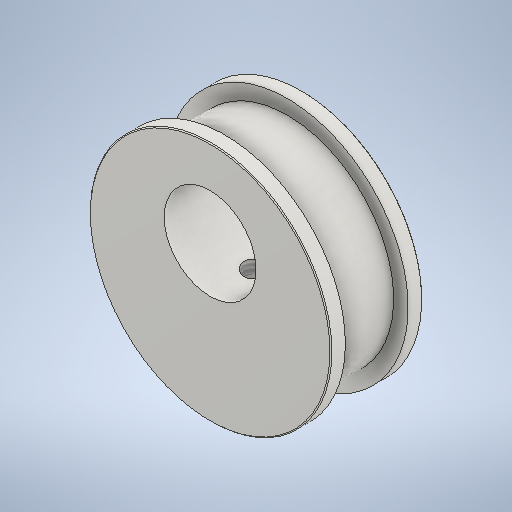
# Autodesk Inventor part: 28 - Eccentric  Sheav
Saved by Autodesk Inventor 2025.2 (Build 292293000, 293)
## iProperties
Created: 2025-07-17
Part Number: 28 - Eccentric  Sheav
Material: Steel AISI 1020 108 ANLD
Document SubType Name: Modeling
Designer: bless
Density: 7.87 g/cm^3
Appearance: Steel
Author: bless
Autodesk Inventor part; units mm, degrees
ref_plane "YZ Plane" through (0, 0, 0) normal (1, 0, 0) x (0, 1, 0)
ref_plane "XZ Plane" through (0, 0, 0) normal (0, 1, 0) x (-1, 0, 0)
ref_plane "XY Plane" through (0, 0, 0) normal (0, 0, 1) x (1, 0, 0)
sketch "Sketch1" plane through (0, 0, 0) normal (0, 0, 1) x (1, 0, 0)
  circle A0 centre (0, 0) radius 12.5
  dimension "d0" = 25
  constraints: 1 centre point, 1 coincident
  measures "d0" diameter of A0
extrude "Extrusion1" add sketch "Sketch1" along normal blind 1.5
sketch "Sketch2" plane through (0, 0, 0) normal (0, 0, -1) x (-1, 0, 0)
  circle A0 centre (0, 0) radius 12.5 projected
  circle A1 centre (0, 0) radius 11
  dimension "d3" = 22
  constraints: 1 centre point, 1 coincident
  measures "d3" diameter of A1
extrude "Extrusion2" add sketch "Sketch2" along normal blind 6.5 contours A1
sketch "Sketch3" plane through (0, 0, -6.5) normal (0, 0, -1) x (-1, 0, 0)
  circle A0 centre (0, 0) radius 11 projected
  circle A1 centre (0, 0) radius 12.5
  dimension "d6" = 25
  constraints: 1 centre point, 1 coincident
  measures "d6" diameter of A1
extrude "Extrusion3" add sketch "Sketch3" along normal blind 1.5 contours A0 | A1
sketch "Sketch4" plane through (0, 0, -8) normal (0, 0, -1) x (-1, 0, 0)
  circle A0 centre (0, 0) radius 12.5 projected
  circle A1 centre (0, 3.5) radius 4.75
  dimension "d9" = 3.5
  dimension "d10" = 9.5
  constraints: 1 centre point, 1 vertical alignment
  measures "d9" distance of A0.centre A1.centre
  measures "d10" diameter of A1
extrude "Extrusion4" cut sketch "Sketch4" against normal through all contours A1
sketch "Sketch6" plane through (0, 0, 0) normal (0, 1, 0) x (-1, 0, 0)
  line L0 (11, 0) -> (11, -6.5) projected
  line L1 (-11, 0) -> (-11, -6.5) projected
  line L2 (-12.5, -6.5) -> (12.5, -6.5) projected
  point P0 (0, 0)
  point P1 (0, -3.25)
  point P2 (11, -3.25)
  dimension "d18" = 11
  dimension "d19" = 3.25
  constraints: 1 midpoint
  measures "d18" distance of point (11, -3.25) point (0, -3.25)
  measures "d19" distance from line of L2 point (0, -3.25)
hole "Hole1" at (0, 0, -3.25) direction (0, -1, 0) diameter 2.459 end through all thread size "M3x0.5" class "6H" standard "ANSI Metric M Profile"
chamfer "Chamfer1" distance 0.1 angle 45 2 edges at (12.5, 0, -8) (-12.5, 0, 1.5)
body "Solid1"
